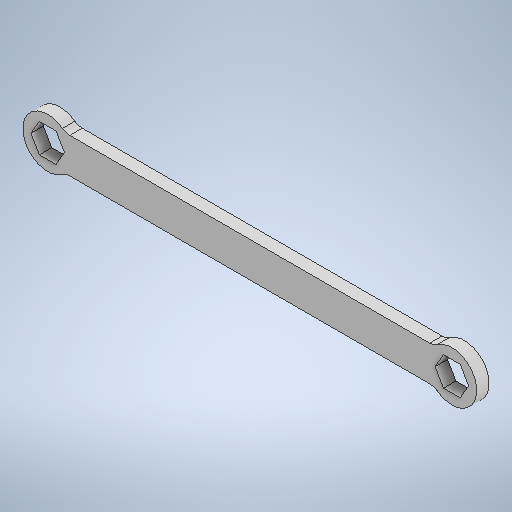
# Autodesk Inventor part: 2P.03.01.15.ZW.FlapCoupler
Saved by Autodesk Inventor 2025.2 (Build 292293000, 293)
## iProperties
Created: 2025-01-14
Part Number: 2P.03.01.15.ZW.FlapCoupler
Material: Generic
Document SubType Name: Modeling
Designer: Imist
Density: 1 g/cm^3
Appearance: Default
Author: Imist
Autodesk Inventor part; units mm, degrees
ref_plane "YZ Plane" through (0, 0, 0) normal (1, 0, 0) x (0, 1, 0)
ref_plane "XZ Plane" through (0, 0, 0) normal (0, 1, 0) x (-1, 0, 0)
ref_plane "XY Plane" through (0, 0, 0) normal (0, 0, 1) x (1, 0, 0)
sketch "Sketch1" plane through (0, 0, 0) normal (0, 0, 1) x (1, 0, 0)
  circle A0 centre (-48.7867, 0.1109) radius 3.5
  circle A1 centre (48.7423, 0.1109) radius 3.5
  arc A2 (-48.7867, 6.1109) -> (-48.7867, -5.8891) centre (-48.7867, 0.1109) ccw
  arc A3 (48.7423, -5.8891) -> (48.7423, 6.1109) centre (48.7423, 0.1109) ccw
  arc A4 (-48.7867, -5.8891) -> (-45.2249, -4.7176) centre (-48.7867, 0.1109) ccw
  line L0 (-48.7867, 0.1109) -> (-44.544, -4.1318) construction
  line L1 (-48.7867, 0.1109) -> (-48.7867, -5.8891) construction
  arc A5 (-45.2249, 4.9393) -> (-48.7867, 6.1109) centre (-48.7867, 0.1109) ccw
  line L2 (-48.7867, 0.1109) -> (-44.544, 4.3535) construction
  line L3 (-48.7867, 0.1109) -> (-48.7867, 6.1109) construction
  arc A6 (48.7423, 6.1109) -> (45.1805, 4.9393) centre (48.7423, 0.1109) ccw
  line L4 (48.7423, 0.1109) -> (44.4997, 4.3535) construction
  line L5 (48.7423, 0.1109) -> (48.7423, 6.1109) construction
  arc A7 (45.1805, -4.7176) -> (48.7423, -5.8891) centre (48.7423, 0.1109) ccw
  line L6 (48.7423, 0.1109) -> (44.4997, -4.1318) construction
  line L7 (48.7423, 0.1109) -> (48.7423, -5.8891) construction
  line L8 (-43.444, 4.3535) -> (43.3997, 4.3535)
  line L9 (-43.444, -4.1318) -> (43.3997, -4.1318)
  arc A8 (-45.2249, 4.9393) -> (-43.444, 4.3535) centre (-43.444, 7.3535) ccw
  arc A9 (-43.444, -4.1318) -> (-45.2249, -4.7176) centre (-43.444, -7.1318) ccw
  arc A10 (43.3997, 4.3535) -> (45.1805, 4.9393) centre (43.3997, 7.3535) ccw
  arc A11 (45.1805, -4.7176) -> (43.3997, -4.1318) centre (43.3997, -7.1318) ccw
  line L10 (-44.7452, 0.1109) -> (-46.7659, -3.3891)
  line L11 (-46.7659, -3.3891) -> (-50.8074, -3.3891)
  line L12 (-50.8074, -3.3891) -> (-52.8281, 0.1109)
  line L13 (-52.8281, 0.1109) -> (-50.8074, 3.6109)
  line L14 (-50.8074, 3.6109) -> (-46.7659, 3.6109)
  line L15 (-46.7659, 3.6109) -> (-44.7452, 0.1109)
  line L16 (44.7009, 0.1109) -> (46.7216, 3.6109)
  line L17 (46.7216, 3.6109) -> (50.7631, 3.6109)
  line L18 (50.7631, 3.6109) -> (52.7838, 0.1109)
  line L19 (52.7838, 0.1109) -> (50.7631, -3.3891)
  line L20 (50.7631, -3.3891) -> (46.7216, -3.3891)
  line L21 (46.7216, -3.3891) -> (44.7009, 0.1109)
  point P0 (0, 0)
  point P1 (44.4997, 4.3535)
  dimension "d0" = 7
  dimension "d1" = 7
  dimension "d2" = 97.529
  dimension "d3" = 6
  dimension "d4" = 6
  dimension "d5" = 45
  dimension "d6" = 45
  dimension "d7" = 45
  dimension "d8" = 45
  dimension "d9" = 3
  constraints: 44 end point, 24 point on circle, 12 centre point, 10 tangent, 9 coincident, 4 point on line, 3 equal radius, 1 horizontal, 26 other
  measures "d0" diameter of A0
  measures "d1" diameter of A1
  measures "d2" distance of L1.end L7.end
  measures "d3" radius of A2
  measures "d4" radius of A3
  measures "d5" angle of L1 L0
  measures "d6" angle of L2 L3
  measures "d7" angle of L5 L4
  measures "d8" angle of L6 L7
  measures "d9" radius of A8
extrude "Extrusion2" add sketch "Sketch1" along normal blind 3
body "Solid2"
